Autodesk Fusion 360 part; units mm, degrees
(part 3 of 5)
sketch "Sketch12" plane through (0, 0, -0.05) normal (0, 0, -1) x (1, 0, 0)
  arc A0 (182.0197, 37.184) -> (182.1217, 37.286) centre (182.0197, 37.286) ccw
  line L0 (182.0197, 37.184) -> (180.0197, 37.184)
  arc A1 (179.9177, 37.286) -> (180.0197, 37.184) centre (180.0197, 37.286) ccw
  line L1 (179.9177, 37.286) -> (179.9177, 38.794)
  arc A2 (180.0197, 38.896) -> (179.9177, 38.794) centre (180.0197, 38.794) ccw
  line L2 (180.0197, 38.896) -> (182.0197, 38.896)
  arc A3 (182.1217, 38.794) -> (182.0197, 38.896) centre (182.0197, 38.794) ccw
  line L3 (182.1217, 38.794) -> (182.1217, 37.286)
  arc A4 (164.6322, 37.184) -> (164.7342, 37.286) centre (164.6322, 37.286) ccw
  line L4 (164.6322, 37.184) -> (162.6322, 37.184)
  arc A5 (162.5302, 37.286) -> (162.6322, 37.184) centre (162.6322, 37.286) ccw
  line L5 (162.5302, 37.286) -> (162.5302, 38.794)
  arc A6 (162.6322, 38.896) -> (162.5302, 38.794) centre (162.6322, 38.794) ccw
  line L6 (162.6322, 38.896) -> (164.6322, 38.896)
  arc A7 (164.7342, 38.794) -> (164.6322, 38.896) centre (164.6322, 38.794) ccw
  line L7 (164.7342, 38.794) -> (164.7342, 37.286)
  line L8 (154.86, 40.74) -> (154.86, 38.54)
  line L9 (154.86, 38.54) -> (153.66, 38.54)
  line L10 (153.66, 38.54) -> (153.66, 40.74)
  line L11 (153.66, 40.74) -> (154.86, 40.74)
  line L12 (139.26, 40.74) -> (139.26, 38.54)
  line L13 (139.26, 38.54) -> (138.06, 38.54)
  line L14 (138.06, 38.54) -> (138.06, 40.74)
  line L15 (138.06, 40.74) -> (139.26, 40.74)
  arc A8 (182.0197, 39.724) -> (182.1217, 39.826) centre (182.0197, 39.826) ccw
  line L16 (182.0197, 39.724) -> (180.0197, 39.724)
  arc A9 (179.9177, 39.826) -> (180.0197, 39.724) centre (180.0197, 39.826) ccw
  line L17 (179.9177, 39.826) -> (179.9177, 41.334)
  arc A10 (180.0197, 41.436) -> (179.9177, 41.334) centre (180.0197, 41.334) ccw
  line L18 (180.0197, 41.436) -> (182.0197, 41.436)
  arc A11 (182.1217, 41.334) -> (182.0197, 41.436) centre (182.0197, 41.334) ccw
  line L19 (182.1217, 41.334) -> (182.1217, 39.826)
  arc A12 (164.6322, 39.724) -> (164.7342, 39.826) centre (164.6322, 39.826) ccw
  line L20 (164.6322, 39.724) -> (162.6322, 39.724)
  arc A13 (162.5302, 39.826) -> (162.6322, 39.724) centre (162.6322, 39.826) ccw
  line L21 (162.5302, 39.826) -> (162.5302, 41.334)
  arc A14 (162.6322, 41.436) -> (162.5302, 41.334) centre (162.6322, 41.334) ccw
  line L22 (162.6322, 41.436) -> (164.6322, 41.436)
  arc A15 (164.7342, 41.334) -> (164.6322, 41.436) centre (164.6322, 41.334) ccw
  line L23 (164.7342, 41.334) -> (164.7342, 39.826)
  circle A16 centre (210.09, 40.19) radius 1.3
  circle A17 centre (129.53, 40.19) radius 1.3
  arc A18 (182.0197, 42.264) -> (182.1217, 42.366) centre (182.0197, 42.366) ccw
  line L24 (182.0197, 42.264) -> (180.0197, 42.264)
  arc A19 (179.9177, 42.366) -> (180.0197, 42.264) centre (180.0197, 42.366) ccw
  line L25 (179.9177, 42.366) -> (179.9177, 43.874)
  arc A20 (180.0197, 43.976) -> (179.9177, 43.874) centre (180.0197, 43.874) ccw
  line L26 (180.0197, 43.976) -> (182.0197, 43.976)
  arc A21 (182.1217, 43.874) -> (182.0197, 43.976) centre (182.0197, 43.874) ccw
  line L27 (182.1217, 43.874) -> (182.1217, 42.366)
  arc A22 (164.6322, 42.264) -> (164.7342, 42.366) centre (164.6322, 42.366) ccw
  line L28 (164.6322, 42.264) -> (162.6322, 42.264)
  arc A23 (162.5302, 42.366) -> (162.6322, 42.264) centre (162.6322, 42.366) ccw
  line L29 (162.5302, 42.366) -> (162.5302, 43.874)
  arc A24 (162.6322, 43.976) -> (162.5302, 43.874) centre (162.6322, 43.874) ccw
  line L30 (162.6322, 43.976) -> (164.6322, 43.976)
  arc A25 (164.7342, 43.874) -> (164.6322, 43.976) centre (164.6322, 43.874) ccw
  line L31 (164.7342, 43.874) -> (164.7342, 42.366)
  circle A26 centre (211.58, 45.04) radius 0.85
  arc A27 (182.0197, 44.804) -> (182.1217, 44.906) centre (182.0197, 44.906) ccw
  line L32 (182.0197, 44.804) -> (180.0197, 44.804)
  arc A28 (179.9177, 44.906) -> (180.0197, 44.804) centre (180.0197, 44.906) ccw
  line L33 (179.9177, 44.906) -> (179.9177, 46.414)
  arc A29 (180.0197, 46.516) -> (179.9177, 46.414) centre (180.0197, 46.414) ccw
  line L34 (180.0197, 46.516) -> (182.0197, 46.516)
  arc A30 (182.1217, 46.414) -> (182.0197, 46.516) centre (182.0197, 46.414) ccw
  line L35 (182.1217, 46.414) -> (182.1217, 44.906)
  arc A31 (164.6322, 44.804) -> (164.7342, 44.906) centre (164.6322, 44.906) ccw
  line L36 (164.6322, 44.804) -> (162.6322, 44.804)
  arc A32 (162.5302, 44.906) -> (162.6322, 44.804) centre (162.6322, 44.906) ccw
  line L37 (162.5302, 44.906) -> (162.5302, 46.414)
  arc A33 (162.6322, 46.516) -> (162.5302, 46.414) centre (162.6322, 46.414) ccw
  line L38 (162.6322, 46.516) -> (164.6322, 46.516)
  arc A34 (164.7342, 46.414) -> (164.6322, 46.516) centre (164.6322, 46.414) ccw
  line L39 (164.7342, 46.414) -> (164.7342, 44.906)
  circle A35 centre (201.97, 46.1501) radius 0.6604
  circle A36 centre (199.43, 46.1501) radius 0.6604
  circle A37 centre (196.89, 46.1501) radius 0.6604
  circle A38 centre (211.58, 47.58) radius 0.85
  arc A39 (182.0197, 47.344) -> (182.1217, 47.446) centre (182.0197, 47.446) ccw
  line L40 (182.0197, 47.344) -> (180.0197, 47.344)
  arc A40 (179.9177, 47.446) -> (180.0197, 47.344) centre (180.0197, 47.446) ccw
  line L41 (179.9177, 47.446) -> (179.9177, 48.954)
  arc A41 (180.0197, 49.056) -> (179.9177, 48.954) centre (180.0197, 48.954) ccw
  line L42 (180.0197, 49.056) -> (182.0197, 49.056)
  arc A42 (182.1217, 48.954) -> (182.0197, 49.056) centre (182.0197, 48.954) ccw
  line L43 (182.1217, 48.954) -> (182.1217, 47.446)
  arc A43 (164.6322, 47.344) -> (164.7342, 47.446) centre (164.6322, 47.446) ccw
  line L44 (164.6322, 47.344) -> (162.6322, 47.344)
  arc A44 (162.5302, 47.446) -> (162.6322, 47.344) centre (162.6322, 47.446) ccw
  line L45 (162.5302, 47.446) -> (162.5302, 48.954)
  arc A45 (162.6322, 49.056) -> (162.5302, 48.954) centre (162.6322, 48.954) ccw
  line L46 (162.6322, 49.056) -> (164.6322, 49.056)
  arc A46 (164.7342, 48.954) -> (164.6322, 49.056) centre (164.6322, 48.954) ccw
  line L47 (164.7342, 48.954) -> (164.7342, 47.446)
  line L48 (154.11, 49.99) -> (154.11, 48.49)
  line L49 (154.11, 48.49) -> (152.51, 48.49)
  line L50 (152.51, 48.49) -> (152.51, 49.99)
  line L51 (152.51, 49.99) -> (154.11, 49.99)
  line L52 (139.26, 49.99) -> (139.26, 48.49)
  line L53 (139.26, 48.49) -> (138.06, 48.49)
  line L54 (138.06, 48.49) -> (138.06, 49.99)
  line L55 (138.06, 49.99) -> (139.26, 49.99)
  circle A47 centre (211.58, 50.12) radius 0.85
  line L56 (149.06, 51.04) -> (149.06, 49.44)
  line L57 (149.06, 49.44) -> (148.36, 49.44)
  line L58 (148.36, 49.44) -> (148.36, 51.04)
  line L59 (148.36, 51.04) -> (149.06, 51.04)
  line L60 (147.96, 51.04) -> (147.96, 49.44)
  line L61 (147.96, 49.44) -> (147.26, 49.44)
  line L62 (147.26, 49.44) -> (147.26, 51.04)
  line L63 (147.26, 51.04) -> (147.96, 51.04)
  line L64 (146.86, 51.04) -> (146.86, 49.44)
  line L65 (146.86, 49.44) -> (146.16, 49.44)
  line L66 (146.16, 49.44) -> (146.16, 51.04)
  line L67 (146.16, 51.04) -> (146.86, 51.04)
  line L68 (145.76, 51.04) -> (145.76, 49.44)
  line L69 (145.76, 49.44) -> (145.06, 49.44)
  line L70 (145.06, 49.44) -> (145.06, 51.04)
  line L71 (145.06, 51.04) -> (145.76, 51.04)
  line L72 (144.66, 51.04) -> (144.66, 49.44)
  line L73 (144.66, 49.44) -> (143.96, 49.44)
  line L74 (143.96, 49.44) -> (143.96, 51.04)
  line L75 (143.96, 51.04) -> (144.66, 51.04)
  line L76 (143.56, 51.04) -> (143.56, 49.44)
  line L77 (143.56, 49.44) -> (142.86, 49.44)
  line L78 (142.86, 49.44) -> (142.86, 51.04)
  line L79 (142.86, 51.04) -> (143.56, 51.04)
  line L80 (142.46, 51.04) -> (142.46, 49.44)
  line L81 (142.46, 49.44) -> (141.76, 49.44)
  line L82 (141.76, 49.44) -> (141.76, 51.04)
  line L83 (141.76, 51.04) -> (142.46, 51.04)
  line L84 (141.36, 51.04) -> (141.36, 49.44)
  line L85 (141.36, 49.44) -> (140.66, 49.44)
  line L86 (140.66, 49.44) -> (140.66, 51.04)
  line L87 (140.66, 51.04) -> (141.36, 51.04)
  line L88 (140.26, 51.04) -> (140.26, 49.44)
  line L89 (140.26, 49.44) -> (139.56, 49.44)
  line L90 (139.56, 49.44) -> (139.56, 51.04)
  line L91 (139.56, 51.04) -> (140.26, 51.04)
  arc A48 (182.0197, 49.884) -> (182.1217, 49.986) centre (182.0197, 49.986) ccw
  line L92 (182.0197, 49.884) -> (180.0197, 49.884)
  arc A49 (179.9177, 49.986) -> (180.0197, 49.884) centre (180.0197, 49.986) ccw
  line L93 (179.9177, 49.986) -> (179.9177, 51.494)
  arc A50 (180.0197, 51.596) -> (179.9177, 51.494) centre (180.0197, 51.494) ccw
  line L94 (180.0197, 51.596) -> (182.0197, 51.596)
  arc A51 (182.1217, 51.494) -> (182.0197, 51.596) centre (182.0197, 51.494) ccw
  line L95 (182.1217, 51.494) -> (182.1217, 49.986)
  arc A52 (164.6322, 49.884) -> (164.7342, 49.986) centre (164.6322, 49.986) ccw
  line L96 (164.6322, 49.884) -> (162.6322, 49.884)
  arc A53 (162.5302, 49.986) -> (162.6322, 49.884) centre (162.6322, 49.986) ccw
  line L97 (162.5302, 49.986) -> (162.5302, 51.494)
  arc A54 (162.6322, 51.596) -> (162.5302, 51.494) centre (162.6322, 51.494) ccw
  line L98 (162.6322, 51.596) -> (164.6322, 51.596)
  arc A55 (164.7342, 51.494) -> (164.6322, 51.596) centre (164.6322, 51.494) ccw
  line L99 (164.7342, 51.494) -> (164.7342, 49.986)
  circle A56 centre (211.58, 52.66) radius 0.85
  arc A57 (182.0197, 52.424) -> (182.1217, 52.526) centre (182.0197, 52.526) ccw
  line L100 (182.0197, 52.424) -> (180.0197, 52.424)
  arc A58 (179.9177, 52.526) -> (180.0197, 52.424) centre (180.0197, 52.526) ccw
  line L101 (179.9177, 52.526) -> (179.9177, 54.034)
  arc A59 (180.0197, 54.136) -> (179.9177, 54.034) centre (180.0197, 54.034) ccw
  line L102 (180.0197, 54.136) -> (182.0197, 54.136)
  arc A60 (182.1217, 54.034) -> (182.0197, 54.136) centre (182.0197, 54.034) ccw
  line L103 (182.1217, 54.034) -> (182.1217, 52.526)
  arc A61 (164.6322, 52.424) -> (164.7342, 52.526) centre (164.6322, 52.526) ccw
  line L104 (164.6322, 52.424) -> (162.6322, 52.424)
  arc A62 (162.5302, 52.526) -> (162.6322, 52.424) centre (162.6322, 52.526) ccw
  line L105 (162.5302, 52.526) -> (162.5302, 54.034)
  arc A63 (162.6322, 54.136) -> (162.5302, 54.034) centre (162.6322, 54.034) ccw
  line L106 (162.6322, 54.136) -> (164.6322, 54.136)
  arc A64 (164.7342, 54.034) -> (164.6322, 54.136) centre (164.6322, 54.034) ccw
  line L107 (164.7342, 54.034) -> (164.7342, 52.526)
  arc A65 (202.19, 52.73) -> (202.44, 52.98) centre (202.19, 52.98) ccw
  line L108 (202.19, 52.73) -> (201.54, 52.73)
  arc A66 (201.29, 52.98) -> (201.54, 52.73) centre (201.54, 52.98) ccw
  line L109 (201.29, 52.98) -> (201.29, 54.28)
  arc A67 (201.54, 54.53) -> (201.29, 54.28) centre (201.54, 54.28) ccw
  line L110 (201.54, 54.53) -> (202.19, 54.53)
  arc A68 (202.44, 54.28) -> (202.19, 54.53) centre (202.19, 54.28) ccw
  line L111 (202.44, 54.28) -> (202.44, 52.98)
  arc A69 (199.24, 52.73) -> (199.49, 52.98) centre (199.24, 52.98) ccw
  line L112 (199.24, 52.73) -> (198.59, 52.73)
  arc A70 (198.34, 52.98) -> (198.59, 52.73) centre (198.59, 52.98) ccw
  line L113 (198.34, 52.98) -> (198.34, 54.28)
  arc A71 (198.59, 54.53) -> (198.34, 54.28) centre (198.59, 54.28) ccw
  line L114 (198.59, 54.53) -> (199.24, 54.53)
  arc A72 (199.49, 54.28) -> (199.24, 54.53) centre (199.24, 54.28) ccw
  line L115 (199.49, 54.28) -> (199.49, 52.98)
  circle A73 centre (211.58, 55.2) radius 0.85
  arc A74 (182.0197, 54.964) -> (182.1217, 55.066) centre (182.0197, 55.066) ccw
  line L116 (182.0197, 54.964) -> (180.0197, 54.964)
  arc A75 (179.9177, 55.066) -> (180.0197, 54.964) centre (180.0197, 55.066) ccw
  line L117 (179.9177, 55.066) -> (179.9177, 56.574)
  arc A76 (180.0197, 56.676) -> (179.9177, 56.574) centre (180.0197, 56.574) ccw
  line L118 (180.0197, 56.676) -> (182.0197, 56.676)
  arc A77 (182.1217, 56.574) -> (182.0197, 56.676) centre (182.0197, 56.574) ccw
  line L119 (182.1217, 56.574) -> (182.1217, 55.066)
  arc A78 (164.6322, 54.964) -> (164.7342, 55.066) centre (164.6322, 55.066) ccw
  line L120 (164.6322, 54.964) -> (162.6322, 54.964)
  arc A79 (162.5302, 55.066) -> (162.6322, 54.964) centre (162.6322, 55.066) ccw
  line L121 (162.5302, 55.066) -> (162.5302, 56.574)
  arc A80 (162.6322, 56.676) -> (162.5302, 56.574) centre (162.6322, 56.574) ccw
  line L122 (162.6322, 56.676) -> (164.6322, 56.676)
  arc A81 (164.7342, 56.574) -> (164.6322, 56.676) centre (164.6322, 56.574) ccw
  line L123 (164.7342, 56.574) -> (164.7342, 55.066)
  circle A82 centre (211.58, 57.74) radius 0.85
  arc A83 (182.0197, 57.504) -> (182.1217, 57.606) centre (182.0197, 57.606) ccw
  line L124 (182.0197, 57.504) -> (180.0197, 57.504)
  arc A84 (179.9177, 57.606) -> (180.0197, 57.504) centre (180.0197, 57.606) ccw
  line L125 (179.9177, 57.606) -> (179.9177, 59.114)
  arc A85 (180.0197, 59.216) -> (179.9177, 59.114) centre (180.0197, 59.114) ccw
  line L126 (180.0197, 59.216) -> (182.0197, 59.216)
  arc A86 (182.1217, 59.114) -> (182.0197, 59.216) centre (182.0197, 59.114) ccw
  line L127 (182.1217, 59.114) -> (182.1217, 57.606)
  arc A87 (164.6391, 57.504) -> (164.7411, 57.606) centre (164.6391, 57.606) ccw
  line L128 (164.6391, 57.504) -> (162.6391, 57.504)
  arc A88 (162.5371, 57.606) -> (162.6391, 57.504) centre (162.6391, 57.606) ccw
  line L129 (162.5371, 57.606) -> (162.5371, 59.114)
  arc A89 (162.6391, 59.216) -> (162.5371, 59.114) centre (162.6391, 59.114) ccw
  line L130 (162.6391, 59.216) -> (164.6391, 59.216)
  arc A90 (164.7411, 59.114) -> (164.6391, 59.216) centre (164.6391, 59.114) ccw
  line L131 (164.7411, 59.114) -> (164.7411, 57.606)
  circle A91 centre (211.58, 60.28) radius 0.85
  circle A92 centre (211.58, 62.82) radius 0.85
  circle A93 centre (211.58, 65.36) radius 0.85
  circle A94 centre (211.58, 67.9) radius 0.85
  circle A95 centre (211.58, 70.44) radius 0.85
  circle A96 centre (211.58, 72.98) radius 0.85
  circle A97 centre (211.58, 75.52) radius 0.85
  line L132 (212.43, 78.91) -> (212.43, 77.21)
  line L133 (212.43, 77.21) -> (210.73, 77.21)
  line L134 (210.73, 77.21) -> (210.73, 78.91)
  line L135 (210.73, 78.91) -> (212.43, 78.91)
  circle A98 centre (184.5, 98.08) radius 1.077
  arc A99 (172.975, 97.003) -> (173.077, 97.105) centre (172.975, 97.105) ccw
  line L136 (172.975, 97.003) -> (171.025, 97.003)
  arc A100 (170.923, 97.105) -> (171.025, 97.003) centre (171.025, 97.105) ccw
  line L137 (170.923, 97.105) -> (170.923, 99.055)
  arc A101 (171.025, 99.157) -> (170.923, 99.055) centre (171.025, 99.055) ccw
  line L138 (171.025, 99.157) -> (172.975, 99.157)
  arc A102 (173.077, 99.055) -> (172.975, 99.157) centre (172.975, 99.055) ccw
  line L139 (173.077, 99.055) -> (173.077, 97.105)
  circle A103 centre (210.09, 102.8) radius 1.3
  circle A104 centre (129.53, 102.8) radius 1.3
  circle A105 centre (184.5, 103.08) radius 1.077
  circle A106 centre (172, 103.08) radius 1.077
  line L140 (205.7384, 36.19) -> (205.7384, 35.19)
  line L141 (205.7384, 35.19) -> (210.09, 35.19)
  line L142 (210.09, 35.19) -> (210.3082, 35.1924)
  arc A107 (210.3082, 35.1924) -> (215.0876, 39.9718) centre (210.09, 40.19) ccw
  line L143 (215.0876, 39.9718) -> (215.09, 40.19)
  line L144 (215.09, 40.19) -> (215.09, 102.8)
  line L145 (215.09, 102.8) -> (215.0877, 103.0182)
  arc A108 (215.0877, 103.0182) -> (210.3082, 107.7977) centre (210.09, 102.8) ccw
  line L146 (210.3082, 107.7977) -> (210.09, 107.8)
  line L147 (210.09, 107.8) -> (129.53, 107.8)
  line L148 (129.53, 107.8) -> (129.3118, 107.7977)
  arc A109 (129.3118, 107.7977) -> (124.5323, 103.0182) centre (129.53, 102.8) ccw
  line L149 (124.5323, 103.0182) -> (124.53, 102.8)
  line L150 (124.53, 102.8) -> (124.53, 40.19)
  line L151 (124.53, 40.19) -> (124.5324, 39.9718)
  arc A110 (124.5324, 39.9718) -> (129.3118, 35.1924) centre (129.53, 40.19) ccw
  line L152 (129.3118, 35.1924) -> (129.53, 35.19)
  line L153 (129.53, 35.19) -> (193.2554, 35.19)
  line L154 (193.2554, 35.19) -> (193.2554, 36.19)
  line L155 (193.2554, 36.19) -> (205.7384, 36.19)
  circle A111 centre (129.53, 40.19) radius 6.4454
  constraint concentric A17 A111
extrude "Extrude12" add sketch "Sketch12" along normal blind 20.4 contours A17 | L150 L151 A110 L152 L153 A111 picked at (125.8386, 41.7899)
sketch "Sketch13" plane through (0, 0, 1.56) normal (0, 0, 1) x (-1, 0, 0)
  arc A0 (-129.3118, 35.1924) -> (-124.5324, 39.9718) centre (-129.53, 40.19) ccw
  line L0 (-124.5324, 39.9718) -> (-124.53, 40.19)
  line L1 (-124.53, 40.19) -> (-124.53, 102.8)
  line L2 (-124.53, 102.8) -> (-124.5323, 103.0182)
  arc A1 (-124.5323, 103.0182) -> (-129.3118, 107.7977) centre (-129.53, 102.8) ccw
  line L3 (-129.3118, 107.7977) -> (-129.53, 107.8)
  line L4 (-129.53, 107.8) -> (-210.09, 107.8)
  line L5 (-210.09, 107.8) -> (-210.3082, 107.7977)
  arc A2 (-210.3082, 107.7977) -> (-215.0877, 103.0182) centre (-210.09, 102.8) ccw
  line L6 (-215.0877, 103.0182) -> (-215.09, 102.8)
  line L7 (-215.09, 102.8) -> (-215.09, 40.19)
  line L8 (-215.09, 40.19) -> (-215.0876, 39.9718)
  arc A3 (-215.0876, 39.9718) -> (-210.3082, 35.1924) centre (-210.09, 40.19) ccw
  line L9 (-210.3082, 35.1924) -> (-210.09, 35.19)
  line L10 (-210.09, 35.19) -> (-129.53, 35.19)
  line L11 (-129.53, 35.19) -> (-129.3118, 35.1924)
  circle A4 centre (-129.53, 102.8) radius 2.2
  circle A5 centre (-210.09, 102.8) radius 2.2
  line L12 (-153, 103.32) -> (-153, 104.72)
  line L13 (-153, 104.72) -> (-151, 104.72)
  line L14 (-151, 104.72) -> (-151, 103.32)
  line L15 (-151, 103.32) -> (-153, 103.32)
  line L16 (-164.46, 103.32) -> (-164.46, 104.72)
  line L17 (-164.46, 104.72) -> (-162.46, 104.72)
  line L18 (-162.46, 104.72) -> (-162.46, 103.32)
  line L19 (-162.46, 103.32) -> (-164.46, 103.32)
  circle A6 centre (-172, 103.08) radius 1.077
  circle A7 centre (-184.5, 103.08) radius 1.077
  line L20 (-153, 100.52) -> (-153, 101.92)
  line L21 (-153, 101.92) -> (-151, 101.92)
  line L22 (-151, 101.92) -> (-151, 100.52)
  line L23 (-151, 100.52) -> (-153, 100.52)
  line L24 (-164.46, 100.52) -> (-164.46, 101.92)
  line L25 (-164.46, 101.92) -> (-162.46, 101.92)
  line L26 (-162.46, 101.92) -> (-162.46, 100.52)
  line L27 (-162.46, 100.52) -> (-164.46, 100.52)
  arc A8 (-173.077, 97.105) -> (-172.975, 97.003) centre (-172.975, 97.105) ccw
  line L28 (-173.077, 97.105) -> (-173.077, 99.055)
  arc A9 (-172.975, 99.157) -> (-173.077, 99.055) centre (-172.975, 99.055) ccw
  line L29 (-172.975, 99.157) -> (-171.025, 99.157)
  arc A10 (-170.923, 99.055) -> (-171.025, 99.157) centre (-171.025, 99.055) ccw
  line L30 (-170.923, 99.055) -> (-170.923, 97.105)
  arc A11 (-171.025, 97.003) -> (-170.923, 97.105) centre (-171.025, 97.105) ccw
  line L31 (-171.025, 97.003) -> (-172.975, 97.003)
  circle A12 centre (-184.5, 98.08) radius 1.077
  line L32 (-153, 96.82) -> (-153, 98.22)
  line L33 (-153, 98.22) -> (-151, 98.22)
  line L34 (-151, 98.22) -> (-151, 96.82)
  line L35 (-151, 96.82) -> (-153, 96.82)
  line L36 (-164.46, 96.82) -> (-164.46, 98.22)
  line L37 (-164.46, 98.22) -> (-162.46, 98.22)
  line L38 (-162.46, 98.22) -> (-162.46, 96.82)
  line L39 (-162.46, 96.82) -> (-164.46, 96.82)
  line L40 (-212.43, 77.21) -> (-212.43, 78.91)
  line L41 (-212.43, 78.91) -> (-210.73, 78.91)
  line L42 (-210.73, 78.91) -> (-210.73, 77.21)
  line L43 (-210.73, 77.21) -> (-212.43, 77.21)
  circle A13 centre (-211.58, 75.52) radius 0.85
  circle A14 centre (-211.58, 72.98) radius 0.85
  circle A15 centre (-211.58, 70.44) radius 0.85
  circle A16 centre (-211.58, 67.9) radius 0.85
  circle A17 centre (-211.58, 65.36) radius 0.85
  circle A18 centre (-211.58, 62.82) radius 0.85
  circle A19 centre (-211.58, 60.28) radius 0.85
  circle A20 centre (-211.58, 57.74) radius 0.85
  circle A21 centre (-211.58, 55.2) radius 0.85
  circle A22 centre (-211.58, 52.66) radius 0.85
  circle A23 centre (-211.58, 50.12) radius 0.85
  circle A24 centre (-211.58, 47.58) radius 0.85
  circle A25 centre (-196.89, 46.1501) radius 0.6604
  circle A26 centre (-199.43, 46.1501) radius 0.6604
  circle A27 centre (-201.97, 46.1501) radius 0.6604
  circle A28 centre (-211.58, 45.04) radius 0.85
  circle A29 centre (-129.53, 40.19) radius 2.2
  circle A30 centre (-210.09, 40.19) radius 2.2
  circle A31 centre (-129.53, 40.1904) radius 2.1996
  circle A32 centre (-129.53, 40.1904) radius 1.0621
  dimension "d43" = -1.1375
  constraint tangent A29 A31
extrude "Extrude13" cut sketch "Sketch13" against normal blind 4.5 contours A32
extrude "Extrude14" cut 1 faces at (211.2977, -38.6274, -20.65) along direction (0, 0, 1) blind 21
sketch "Sketch14" plane through (0, 0, -0.05) normal (0, 0, -1) x (1, 0, 0)
  arc A0 (182.0197, 37.184) -> (182.1217, 37.286) centre (182.0197, 37.286) ccw
  line L0 (182.0197, 37.184) -> (180.0197, 37.184)
  arc A1 (179.9177, 37.286) -> (180.0197, 37.184) centre (180.0197, 37.286) ccw
  line L1 (179.9177, 37.286) -> (179.9177, 38.794)
  arc A2 (180.0197, 38.896) -> (179.9177, 38.794) centre (180.0197, 38.794) ccw
  line L2 (180.0197, 38.896) -> (182.0197, 38.896)
  arc A3 (182.1217, 38.794) -> (182.0197, 38.896) centre (182.0197, 38.794) ccw
  line L3 (182.1217, 38.794) -> (182.1217, 37.286)
  arc A4 (164.6322, 37.184) -> (164.7342, 37.286) centre (164.6322, 37.286) ccw
  line L4 (164.6322, 37.184) -> (162.6322, 37.184)
  arc A5 (162.5302, 37.286) -> (162.6322, 37.184) centre (162.6322, 37.286) ccw
  line L5 (162.5302, 37.286) -> (162.5302, 38.794)
  arc A6 (162.6322, 38.896) -> (162.5302, 38.794) centre (162.6322, 38.794) ccw
  line L6 (162.6322, 38.896) -> (164.6322, 38.896)
  arc A7 (164.7342, 38.794) -> (164.6322, 38.896) centre (164.6322, 38.794) ccw
  line L7 (164.7342, 38.794) -> (164.7342, 37.286)
  line L8 (154.86, 40.74) -> (154.86, 38.54)
  line L9 (154.86, 38.54) -> (153.66, 38.54)
  line L10 (153.66, 38.54) -> (153.66, 40.74)
  line L11 (153.66, 40.74) -> (154.86, 40.74)
  line L12 (139.26, 40.74) -> (139.26, 38.54)
  line L13 (139.26, 38.54) -> (138.06, 38.54)
  line L14 (138.06, 38.54) -> (138.06, 40.74)
  line L15 (138.06, 40.74) -> (139.26, 40.74)
  arc A8 (182.0197, 39.724) -> (182.1217, 39.826) centre (182.0197, 39.826) ccw
  line L16 (182.0197, 39.724) -> (180.0197, 39.724)
  arc A9 (179.9177, 39.826) -> (180.0197, 39.724) centre (180.0197, 39.826) ccw
  line L17 (179.9177, 39.826) -> (179.9177, 41.334)
  arc A10 (180.0197, 41.436) -> (179.9177, 41.334) centre (180.0197, 41.334) ccw
  line L18 (180.0197, 41.436) -> (182.0197, 41.436)
  arc A11 (182.1217, 41.334) -> (182.0197, 41.436) centre (182.0197, 41.334) ccw
  line L19 (182.1217, 41.334) -> (182.1217, 39.826)
  arc A12 (164.6322, 39.724) -> (164.7342, 39.826) centre (164.6322, 39.826) ccw
  line L20 (164.6322, 39.724) -> (162.6322, 39.724)
  arc A13 (162.5302, 39.826) -> (162.6322, 39.724) centre (162.6322, 39.826) ccw
  line L21 (162.5302, 39.826) -> (162.5302, 41.334)
  arc A14 (162.6322, 41.436) -> (162.5302, 41.334) centre (162.6322, 41.334) ccw
  line L22 (162.6322, 41.436) -> (164.6322, 41.436)
  arc A15 (164.7342, 41.334) -> (164.6322, 41.436) centre (164.6322, 41.334) ccw
  line L23 (164.7342, 41.334) -> (164.7342, 39.826)
  circle A16 centre (210.09, 40.19) radius 1.3
  circle A17 centre (129.53, 40.19) radius 1.3
  arc A18 (182.0197, 42.264) -> (182.1217, 42.366) centre (182.0197, 42.366) ccw
  line L24 (182.0197, 42.264) -> (180.0197, 42.264)
  arc A19 (179.9177, 42.366) -> (180.0197, 42.264) centre (180.0197, 42.366) ccw
  line L25 (179.9177, 42.366) -> (179.9177, 43.874)
  arc A20 (180.0197, 43.976) -> (179.9177, 43.874) centre (180.0197, 43.874) ccw
  line L26 (180.0197, 43.976) -> (182.0197, 43.976)
  arc A21 (182.1217, 43.874) -> (182.0197, 43.976) centre (182.0197, 43.874) ccw
  line L27 (182.1217, 43.874) -> (182.1217, 42.366)
  arc A22 (164.6322, 42.264) -> (164.7342, 42.366) centre (164.6322, 42.366) ccw
  line L28 (164.6322, 42.264) -> (162.6322, 42.264)
  arc A23 (162.5302, 42.366) -> (162.6322, 42.264) centre (162.6322, 42.366) ccw
  line L29 (162.5302, 42.366) -> (162.5302, 43.874)
  arc A24 (162.6322, 43.976) -> (162.5302, 43.874) centre (162.6322, 43.874) ccw
  line L30 (162.6322, 43.976) -> (164.6322, 43.976)
  arc A25 (164.7342, 43.874) -> (164.6322, 43.976) centre (164.6322, 43.874) ccw
  line L31 (164.7342, 43.874) -> (164.7342, 42.366)
  circle A26 centre (211.58, 45.04) radius 0.85
  arc A27 (182.0197, 44.804) -> (182.1217, 44.906) centre (182.0197, 44.906) ccw
  line L32 (182.0197, 44.804) -> (180.0197, 44.804)
  arc A28 (179.9177, 44.906) -> (180.0197, 44.804) centre (180.0197, 44.906) ccw
  line L33 (179.9177, 44.906) -> (179.9177, 46.414)
  arc A29 (180.0197, 46.516) -> (179.9177, 46.414) centre (180.0197, 46.414) ccw
  line L34 (180.0197, 46.516) -> (182.0197, 46.516)
  arc A30 (182.1217, 46.414) -> (182.0197, 46.516) centre (182.0197, 46.414) ccw
  line L35 (182.1217, 46.414) -> (182.1217, 44.906)
  arc A31 (164.6322, 44.804) -> (164.7342, 44.906) centre (164.6322, 44.906) ccw
  line L36 (164.6322, 44.804) -> (162.6322, 44.804)
  arc A32 (162.5302, 44.906) -> (162.6322, 44.804) centre (162.6322, 44.906) ccw
  line L37 (162.5302, 44.906) -> (162.5302, 46.414)
  arc A33 (162.6322, 46.516) -> (162.5302, 46.414) centre (162.6322, 46.414) ccw
  line L38 (162.6322, 46.516) -> (164.6322, 46.516)
  arc A34 (164.7342, 46.414) -> (164.6322, 46.516) centre (164.6322, 46.414) ccw
  line L39 (164.7342, 46.414) -> (164.7342, 44.906)
  circle A35 centre (201.97, 46.1501) radius 0.6604
  circle A36 centre (199.43, 46.1501) radius 0.6604
  circle A37 centre (196.89, 46.1501) radius 0.6604
  circle A38 centre (211.58, 47.58) radius 0.85
  arc A39 (182.0197, 47.344) -> (182.1217, 47.446) centre (182.0197, 47.446) ccw
  line L40 (182.0197, 47.344) -> (180.0197, 47.344)
  arc A40 (179.9177, 47.446) -> (180.0197, 47.344) centre (180.0197, 47.446) ccw
  line L41 (179.9177, 47.446) -> (179.9177, 48.954)
  arc A41 (180.0197, 49.056) -> (179.9177, 48.954) centre (180.0197, 48.954) ccw
  line L42 (180.0197, 49.056) -> (182.0197, 49.056)
  arc A42 (182.1217, 48.954) -> (182.0197, 49.056) centre (182.0197, 48.954) ccw
  line L43 (182.1217, 48.954) -> (182.1217, 47.446)
  arc A43 (164.6322, 47.344) -> (164.7342, 47.446) centre (164.6322, 47.446) ccw
  line L44 (164.6322, 47.344) -> (162.6322, 47.344)
  arc A44 (162.5302, 47.446) -> (162.6322, 47.344) centre (162.6322, 47.446) ccw
  line L45 (162.5302, 47.446) -> (162.5302, 48.954)
  arc A45 (162.6322, 49.056) -> (162.5302, 48.954) centre (162.6322, 48.954) ccw
  line L46 (162.6322, 49.056) -> (164.6322, 49.056)
  arc A46 (164.7342, 48.954) -> (164.6322, 49.056) centre (164.6322, 48.954) ccw
  line L47 (164.7342, 48.954) -> (164.7342, 47.446)
  line L48 (154.11, 49.99) -> (154.11, 48.49)
  line L49 (154.11, 48.49) -> (152.51, 48.49)
  line L50 (152.51, 48.49) -> (152.51, 49.99)
  line L51 (152.51, 49.99) -> (154.11, 49.99)
  line L52 (139.26, 49.99) -> (139.26, 48.49)
  line L53 (139.26, 48.49) -> (138.06, 48.49)
  line L54 (138.06, 48.49) -> (138.06, 49.99)
  line L55 (138.06, 49.99) -> (139.26, 49.99)
  circle A47 centre (211.58, 50.12) radius 0.85
  line L56 (149.06, 51.04) -> (149.06, 49.44)
  line L57 (149.06, 49.44) -> (148.36, 49.44)
  line L58 (148.36, 49.44) -> (148.36, 51.04)
  line L59 (148.36, 51.04) -> (149.06, 51.04)
  line L60 (147.96, 51.04) -> (147.96, 49.44)
  line L61 (147.96, 49.44) -> (147.26, 49.44)
  line L62 (147.26, 49.44) -> (147.26, 51.04)
  line L63 (147.26, 51.04) -> (147.96, 51.04)
  line L64 (146.86, 51.04) -> (146.86, 49.44)
  line L65 (146.86, 49.44) -> (146.16, 49.44)
  line L66 (146.16, 49.44) -> (146.16, 51.04)
  line L67 (146.16, 51.04) -> (146.86, 51.04)
  line L68 (145.76, 51.04) -> (145.76, 49.44)
  line L69 (145.76, 49.44) -> (145.06, 49.44)
  line L70 (145.06, 49.44) -> (145.06, 51.04)
  line L71 (145.06, 51.04) -> (145.76, 51.04)
  line L72 (144.66, 51.04) -> (144.66, 49.44)
  line L73 (144.66, 49.44) -> (143.96, 49.44)
  line L74 (143.96, 49.44) -> (143.96, 51.04)
  line L75 (143.96, 51.04) -> (144.66, 51.04)
  line L76 (143.56, 51.04) -> (143.56, 49.44)
  line L77 (143.56, 49.44) -> (142.86, 49.44)
  line L78 (142.86, 49.44) -> (142.86, 51.04)
  line L79 (142.86, 51.04) -> (143.56, 51.04)
  line L80 (142.46, 51.04) -> (142.46, 49.44)
  line L81 (142.46, 49.44) -> (141.76, 49.44)
  line L82 (141.76, 49.44) -> (141.76, 51.04)
  line L83 (141.76, 51.04) -> (142.46, 51.04)
  line L84 (141.36, 51.04) -> (141.36, 49.44)
  line L85 (141.36, 49.44) -> (140.66, 49.44)
  line L86 (140.66, 49.44) -> (140.66, 51.04)
  line L87 (140.66, 51.04) -> (141.36, 51.04)
  line L88 (140.26, 51.04) -> (140.26, 49.44)
  line L89 (140.26, 49.44) -> (139.56, 49.44)
  line L90 (139.56, 49.44) -> (139.56, 51.04)
  line L91 (139.56, 51.04) -> (140.26, 51.04)
  arc A48 (182.0197, 49.884) -> (182.1217, 49.986) centre (182.0197, 49.986) ccw
  line L92 (182.0197, 49.884) -> (180.0197, 49.884)
  arc A49 (179.9177, 49.986) -> (180.0197, 49.884) centre (180.0197, 49.986) ccw
  line L93 (179.9177, 49.986) -> (179.9177, 51.494)
  arc A50 (180.0197, 51.596) -> (179.9177, 51.494) centre (180.0197, 51.494) ccw
  line L94 (180.0197, 51.596) -> (182.0197, 51.596)
  arc A51 (182.1217, 51.494) -> (182.0197, 51.596) centre (182.0197, 51.494) ccw
  line L95 (182.1217, 51.494) -> (182.1217, 49.986)
  arc A52 (164.6322, 49.884) -> (164.7342, 49.986) centre (164.6322, 49.986) ccw
  line L96 (164.6322, 49.884) -> (162.6322, 49.884)
  arc A53 (162.5302, 49.986) -> (162.6322, 49.884) centre (162.6322, 49.986) ccw
  line L97 (162.5302, 49.986) -> (162.5302, 51.494)
  arc A54 (162.6322, 51.596) -> (162.5302, 51.494) centre (162.6322, 51.494) ccw
  line L98 (162.6322, 51.596) -> (164.6322, 51.596)
  arc A55 (164.7342, 51.494) -> (164.6322, 51.596) centre (164.6322, 51.494) ccw
  line L99 (164.7342, 51.494) -> (164.7342, 49.986)
  circle A56 centre (211.58, 52.66) radius 0.85
  arc A57 (182.0197, 52.424) -> (182.1217, 52.526) centre (182.0197, 52.526) ccw
  line L100 (182.0197, 52.424) -> (180.0197, 52.424)
  arc A58 (179.9177, 52.526) -> (180.0197, 52.424) centre (180.0197, 52.526) ccw
  line L101 (179.9177, 52.526) -> (179.9177, 54.034)
  arc A59 (180.0197, 54.136) -> (179.9177, 54.034) centre (180.0197, 54.034) ccw
  line L102 (180.0197, 54.136) -> (182.0197, 54.136)
  arc A60 (182.1217, 54.034) -> (182.0197, 54.136) centre (182.0197, 54.034) ccw
  line L103 (182.1217, 54.034) -> (182.1217, 52.526)
  arc A61 (164.6322, 52.424) -> (164.7342, 52.526) centre (164.6322, 52.526) ccw
  line L104 (164.6322, 52.424) -> (162.6322, 52.424)
  arc A62 (162.5302, 52.526) -> (162.6322, 52.424) centre (162.6322, 52.526) ccw
  line L105 (162.5302, 52.526) -> (162.5302, 54.034)
  arc A63 (162.6322, 54.136) -> (162.5302, 54.034) centre (162.6322, 54.034) ccw
  line L106 (162.6322, 54.136) -> (164.6322, 54.136)
  arc A64 (164.7342, 54.034) -> (164.6322, 54.136) centre (164.6322, 54.034) ccw
  line L107 (164.7342, 54.034) -> (164.7342, 52.526)
  arc A65 (202.19, 52.73) -> (202.44, 52.98) centre (202.19, 52.98) ccw
  line L108 (202.19, 52.73) -> (201.54, 52.73)
  arc A66 (201.29, 52.98) -> (201.54, 52.73) centre (201.54, 52.98) ccw
  line L109 (201.29, 52.98) -> (201.29, 54.28)
  arc A67 (201.54, 54.53) -> (201.29, 54.28) centre (201.54, 54.28) ccw
  line L110 (201.54, 54.53) -> (202.19, 54.53)
  arc A68 (202.44, 54.28) -> (202.19, 54.53) centre (202.19, 54.28) ccw
  line L111 (202.44, 54.28) -> (202.44, 52.98)
  arc A69 (199.24, 52.73) -> (199.49, 52.98) centre (199.24, 52.98) ccw
  line L112 (199.24, 52.73) -> (198.59, 52.73)
  arc A70 (198.34, 52.98) -> (198.59, 52.73) centre (198.59, 52.98) ccw
  line L113 (198.34, 52.98) -> (198.34, 54.28)
  arc A71 (198.59, 54.53) -> (198.34, 54.28) centre (198.59, 54.28) ccw
  line L114 (198.59, 54.53) -> (199.24, 54.53)
  arc A72 (199.49, 54.28) -> (199.24, 54.53) centre (199.24, 54.28) ccw
  line L115 (199.49, 54.28) -> (199.49, 52.98)
  circle A73 centre (211.58, 55.2) radius 0.85
  arc A74 (182.0197, 54.964) -> (182.1217, 55.066) centre (182.0197, 55.066) ccw
  line L116 (182.0197, 54.964) -> (180.0197, 54.964)
  arc A75 (179.9177, 55.066) -> (180.0197, 54.964) centre (180.0197, 55.066) ccw
  line L117 (179.9177, 55.066) -> (179.9177, 56.574)
  arc A76 (180.0197, 56.676) -> (179.9177, 56.574) centre (180.0197, 56.574) ccw
  line L118 (180.0197, 56.676) -> (182.0197, 56.676)
  arc A77 (182.1217, 56.574) -> (182.0197, 56.676) centre (182.0197, 56.574) ccw
  line L119 (182.1217, 56.574) -> (182.1217, 55.066)
  arc A78 (164.6322, 54.964) -> (164.7342, 55.066) centre (164.6322, 55.066) ccw
  line L120 (164.6322, 54.964) -> (162.6322, 54.964)
  arc A79 (162.5302, 55.066) -> (162.6322, 54.964) centre (162.6322, 55.066) ccw
  line L121 (162.5302, 55.066) -> (162.5302, 56.574)
  arc A80 (162.6322, 56.676) -> (162.5302, 56.574) centre (162.6322, 56.574) ccw
  line L122 (162.6322, 56.676) -> (164.6322, 56.676)
  arc A81 (164.7342, 56.574) -> (164.6322, 56.676) centre (164.6322, 56.574) ccw
  line L123 (164.7342, 56.574) -> (164.7342, 55.066)
  circle A82 centre (211.58, 57.74) radius 0.85
  arc A83 (182.0197, 57.504) -> (182.1217, 57.606) centre (182.0197, 57.606) ccw
  line L124 (182.0197, 57.504) -> (180.0197, 57.504)
  arc A84 (179.9177, 57.606) -> (180.0197, 57.504) centre (180.0197, 57.606) ccw
  line L125 (179.9177, 57.606) -> (179.9177, 59.114)
  arc A85 (180.0197, 59.216) -> (179.9177, 59.114) centre (180.0197, 59.114) ccw
  line L126 (180.0197, 59.216) -> (182.0197, 59.216)
  arc A86 (182.1217, 59.114) -> (182.0197, 59.216) centre (182.0197, 59.114) ccw
  line L127 (182.1217, 59.114) -> (182.1217, 57.606)
  arc A87 (164.6391, 57.504) -> (164.7411, 57.606) centre (164.6391, 57.606) ccw
  line L128 (164.6391, 57.504) -> (162.6391, 57.504)
  arc A88 (162.5371, 57.606) -> (162.6391, 57.504) centre (162.6391, 57.606) ccw
  line L129 (162.5371, 57.606) -> (162.5371, 59.114)
  arc A89 (162.6391, 59.216) -> (162.5371, 59.114) centre (162.6391, 59.114) ccw
  line L130 (162.6391, 59.216) -> (164.6391, 59.216)
  arc A90 (164.7411, 59.114) -> (164.6391, 59.216) centre (164.6391, 59.114) ccw
  line L131 (164.7411, 59.114) -> (164.7411, 57.606)
  circle A91 centre (211.58, 60.28) radius 0.85
  circle A92 centre (211.58, 62.82) radius 0.85
  circle A93 centre (211.58, 65.36) radius 0.85
  circle A94 centre (211.58, 67.9) radius 0.85
  circle A95 centre (211.58, 70.44) radius 0.85
  circle A96 centre (211.58, 72.98) radius 0.85
  circle A97 centre (211.58, 75.52) radius 0.85
  line L132 (212.43, 78.91) -> (212.43, 77.21)
  line L133 (212.43, 77.21) -> (210.73, 77.21)
  line L134 (210.73, 77.21) -> (210.73, 78.91)
  line L135 (210.73, 78.91) -> (212.43, 78.91)
  circle A98 centre (184.5, 98.08) radius 1.077
  arc A99 (172.975, 97.003) -> (173.077, 97.105) centre (172.975, 97.105) ccw
  line L136 (172.975, 97.003) -> (171.025, 97.003)
  arc A100 (170.923, 97.105) -> (171.025, 97.003) centre (171.025, 97.105) ccw
  line L137 (170.923, 97.105) -> (170.923, 99.055)
  arc A101 (171.025, 99.157) -> (170.923, 99.055) centre (171.025, 99.055) ccw
  line L138 (171.025, 99.157) -> (172.975, 99.157)
  arc A102 (173.077, 99.055) -> (172.975, 99.157) centre (172.975, 99.055) ccw
  line L139 (173.077, 99.055) -> (173.077, 97.105)
  circle A103 centre (210.09, 102.8) radius 1.3
  circle A104 centre (129.53, 102.8) radius 1.3
  circle A105 centre (184.5, 103.08) radius 1.077
  circle A106 centre (172, 103.08) radius 1.077
  line L140 (205.7384, 36.19) -> (205.7384, 35.19)
  line L141 (205.7384, 35.19) -> (210.09, 35.19)
  line L142 (210.09, 35.19) -> (210.3082, 35.1924)
  arc A107 (210.3082, 35.1924) -> (215.0876, 39.9718) centre (210.09, 40.19) ccw
  line L143 (215.0876, 39.9718) -> (215.09, 40.19)
  line L144 (215.09, 40.19) -> (215.09, 102.8)
  line L145 (215.09, 102.8) -> (215.0877, 103.0182)
  arc A108 (215.0877, 103.0182) -> (210.3082, 107.7977) centre (210.09, 102.8) ccw
  line L146 (210.3082, 107.7977) -> (210.09, 107.8)
  line L147 (210.09, 107.8) -> (129.53, 107.8)
  line L148 (129.53, 107.8) -> (129.3118, 107.7977)
  arc A109 (129.3118, 107.7977) -> (124.5323, 103.0182) centre (129.53, 102.8) ccw
  line L149 (124.5323, 103.0182) -> (124.53, 102.8)
  line L150 (124.53, 102.8) -> (124.53, 40.19)
  line L151 (124.53, 40.19) -> (124.5324, 39.9718)
  arc A110 (124.5324, 39.9718) -> (129.3118, 35.1924) centre (129.53, 40.19) ccw
  line L152 (129.3118, 35.1924) -> (129.53, 35.19)
  line L153 (129.53, 35.19) -> (193.2554, 35.19)
  line L154 (193.2554, 35.19) -> (193.2554, 36.19)
  line L155 (193.2554, 36.19) -> (205.7384, 36.19)
  circle A111 centre (211.7385, 38.2976) radius 4.8836
extrude "Extrude15" add sketch "Sketch14" along normal blind 20.4 contours L141 L142 A107 L143 L144 A111 picked at (209.0452, 36.8325)
extrude "Extrude16" cut 1 faces at (129.8072, -102.2176, -20.65) along direction (0, 0, 1) blind 0.2
extrude "Extrude17" cut 1 faces at (209.0452, -36.8325, -20.45) along direction (0, 0, 1) blind 20.5